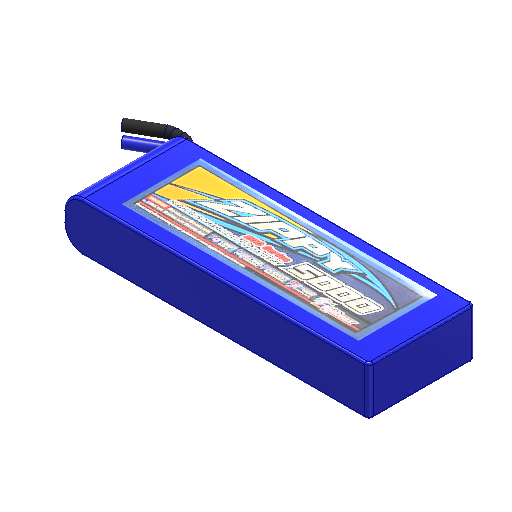
# Autodesk Inventor part: COTS_ZIPPY_Li-Po_Battery_5000mAh_3S
Saved by Autodesk Inventor 2025 (Build 290162010, 162A)
## iProperties
Created: 2017-08-31
Part Number: COTS_ZIPPY_Li-Po_Battery_5000mAh_3S
Material: Ogólny
Document SubType Name: Modeling
Designer: Andrzej
Density: 1 g/cm^3
Appearance: Niebieska - farba ścienna - lśniąca
Mass: 164.189 g
Surface Area: 233.6 cm^2
Volume: 164.189 cm^3
Author: Andrzej
Autodesk Inventor part; units mm, degrees
ref_plane "YZ Plane" through (0, 0, 0) normal (1, 0, 0) x (0, 1, 0)
ref_plane "XZ Plane" through (0, 0, 0) normal (0, 1, 0) x (-1, 0, 0)
ref_plane "XY Plane" through (0, 0, 0) normal (0, 0, 1) x (1, 0, 0)
sketch "Szkic1" plane through (0, 0, 0) normal (0, 0, 1) x (1, 0, 0)
  line L0 (-17.4978, 4.0814) -> (126.0022, 4.0814)
  line L1 (126.0022, 4.0814) -> (126.0022, 54.0814)
  line L2 (126.0022, 54.0814) -> (-17.4978, 54.0814)
  line L3 (-17.4978, 54.0814) -> (-17.4978, 4.0814)
  point P0 (0, 0)
  dimension "d0" = 143.5
  dimension "d1" = 50
  constraints: 8 end point, 2 parallel, 1 horizontal, 1 perpendicular
  measures "d0" distance of L2.end L1.end
  measures "d1" distance of L1.end L0.end
extrude "Wyciągnięcie proste1" add sketch "Szkic1" along normal blind 23
fillet "Zaokrąglenie1" radius 9 2 edges at (-17.4978, 29.0814, 23) (-17.4978, 29.0814, 0)
fillet "Zaokrąglenie2" radius 2 2 edges at (126.0022, 4.0814, 11.5) (126.0022, 54.0814, 11.5)
fillet "Zaokrąglenie3" radius 1 16 edges at (125.4164, 4.6672, 23) (126.0022, 29.0814, 23) (125.4164, 53.4956, 23) (57.7522, 54.0814, 23) (-14.8618, 54.0814, 20.364) (-17.4978, 54.0814, 11.5) (-14.8618, 54.0814, 2.636) (57.7522, 54.0814, 0) (125.4164, 53.4956, 0) (126.0022, 29.0814, 0) (125.4164, 4.6672, 0) (57.7522, 4.0814, 0) (-14.8618, 4.0814, 2.636) (-17.4978, 4.0814, 11.5) (-14.8618, 4.0814, 20.364) (57.7522, 4.0814, 23)
sketch "Szkic2" plane through (0, 0, 23) normal (0, 0, 1) x (1, 0, 0)
  line L0 (2.5572, 48.5476) -> (113.8689, 48.5476) construction
  line L1 (113.8689, 48.5476) -> (113.8689, 11.3084) construction
  line L2 (113.8689, 11.3084) -> (2.5572, 11.3084) construction
  line L3 (2.5572, 11.3084) -> (2.5572, 48.5476) construction
  point P0 (0, 0)
  constraints: 2 other
ref_plane "Płaszczyzna konstrukcyjna1" through (0, 0, 15) normal (0, 0, 1) x (1, 0, 0)
sketch "Szkic3" plane through (0, 0, 15) normal (0, 0, 1) x (1, 0, 0)
  line L0 (-16.4978, 54.0814) -> (-8.4978, 54.0814) projected
  line L1 (-17.4978, 53.0814) -> (-17.4978, 5.0814) projected
  line L2 (-13.4978, 54.0814) -> (-13.4978, 56.0814)
  line L3 (-18.4978, 60.0814) -> (-17.4978, 60.0814)
  arc A0 (-13.4978, 56.0814) -> (-17.4978, 60.0814) centre (-17.4978, 56.0814) ccw
  line L4 (-18.4978, 60.0814) -> (-21.2325, 60.0814)
  line L5 (-24.203, 59.2945) -> (-37.2438, 51.8639)
  arc A1 (-21.2325, 60.0814) -> (-24.203, 59.2945) centre (-21.2325, 54.0814) ccw
  point P0 (0, 0)
  point P1 (-13.4978, 58.0814)
  dimension "d15" = 4
  dimension "d16" = 4
  dimension "d20" = 4
  dimension "d24" = 6
  dimension "d25" = 6
  constraints: 8 end point, 4 point on circle, 4 tangent, 2 centre point, 2 horizontal, 2 point on line, 1 vertical
  measures "d15" distance from line of L2.start L1
  measures "d16" distance of L2.start point (-13.498, 58.081)
  measures "d20" radius of A0
  measures "d24" distance between parallel lines of L0 L3
  measures "d25" radius of A1
sketch "Szkic4" plane through (-8.4978, 54.0814, 1) normal (0, 1, 0) x (1, 0, 0)
  circle A0 centre (-4.9887, -14.0009) radius 2.4
  point P0 (8.4978, 1)
  dimension "d21" = 4.8
  constraints: 1 centre point
  measures "d21" diameter of A0
sweep "Przeciągnięcie1" add profiles "Szkic4" path "Szkic3" path curves L2 A0 L3 L4 A1 L5
pattern_linear "Szyk prostokątny1" count 2 spacing 7 along (0, 0, -1) of "Przeciągnięcie1"
decal "Pokrycie bitmapą1"
